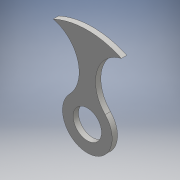
# Autodesk Inventor part: crusher_claw
Saved by Autodesk Inventor 2016 (Build 200138000, 138)
## iProperties
Created: 2016-03-30
Part Number: crusher_claw
Material: Generic
Document SubType Name: Modeling
Designer: 3DPrinterUser
Density: 1 g/cm^3
Appearance: Default
Mass: 0.354461 g
Surface Area: 6.49761 cm^2
Volume: 0.354461 cm^3
Author: 3DPrinterUser
Autodesk Inventor part; units mm, degrees
ref_plane "YZ Plane" through (0, 0, 0) normal (1, 0, 0) x (0, 1, 0)
ref_plane "XZ Plane" through (0, 0, 0) normal (0, 1, 0) x (-1, 0, 0)
ref_plane "XY Plane" through (0, 0, 0) normal (0, 0, 1) x (1, 0, 0)
sketch "Sketch1" plane through (0, 0, 0) normal (0, 1, 0) x (-1, 0, 0)
  circle A0 centre (0, 0) radius 4
  arc A1 (-5.0181, 4.8805) -> (5.0181, 4.8805) centre (0, 0) ccw
  arc A2 (9.6094, 20.8964) -> (-9.6094, 20.8964) centre (0, 0) ccw
  arc A3 (-5.0181, 4.8805) -> (-9.6094, 20.8964) centre (-11.9, 11.5737) ccw
  arc A4 (9.6094, 20.8964) -> (5.0181, 4.8805) centre (11.9, 11.5737) ccw
  line L0 (5.0181, 4.8805) -> (-5.0181, 4.8805)
  dimension "d0" = 8
  dimension "d1" = 14
  dimension "d2" = 46
  dimension "d15" = 9.6
  dimension "d17" = 4.6
  constraints: 8 point on circle, 5 centre point, 3 coincident, 2 end point, 2 tangent, 1 equal radius, 1 horizontal
  measures "d0" diameter of A0
  measures "d1" diameter of A1
  measures "d2" diameter of A2
  measures "d15" radius of A3
extrude "Extrusion3" add sketch "Sketch1" along normal blind 1.5
body "Solid2"
